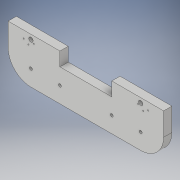
# Autodesk Inventor part: side drivetrain piece (8 wheel macanum)
Saved by Autodesk Inventor 2019 (Build 230136000, 136)
## iProperties
Created: 2019-04-20
Part Number: side drivetrain piece (8 wheel macanum)
Material: Generic
Document SubType Name: Modeling
Designer: Delta
Density: 1 g/cm^3
Appearance: Default
Author: Delta
Autodesk Inventor part; units mm, degrees
ref_plane "YZ Plane" through (0, 0, 0) normal (1, 0, 0) x (0, 1, 0)
ref_plane "XZ Plane" through (0, 0, 0) normal (0, 1, 0) x (-1, 0, 0)
ref_plane "XY Plane" through (0, 0, 0) normal (0, 0, 1) x (1, 0, 0)
sketch "Sketch1" plane through (0, 0, 0) normal (0, 0, 1) x (1, 0, 0)
  line L0 (-63.5, 0) -> (-368.3, 0)
  line L1 (-431.8, 63.5) -> (-431.8, 88.9)
  line L2 (-431.8, 88.9) -> (0, 88.9)
  line L3 (0, 88.9) -> (0, 63.5)
  arc A0 (-431.8, 63.5) -> (-368.3, 0) centre (-368.3, 63.5) ccw
  arc A1 (-63.5, 0) -> (0, 63.5) centre (-63.5, 63.5) ccw
  line L4 (-431.8, 88.9) -> (-287.8667, 88.9)
  line L5 (0, 88.9) -> (-143.9333, 88.9)
  point P0 (0, 0)
  point P1 (-431.8, 0)
  dimension "d0" = 431.8
  dimension "d1" = 88.9
  dimension "d2" = 63.5
  dimension "d3" = 63.5
  constraints: 12 end point, 4 point on circle, 4 point on line, 4 tangent, 3 horizontal, 2 centre point, 2 parallel, 1 perpendicular
  measures "d0" distance of L1.end L2.end
  measures "d1" distance of point (-431.8, 0) L1.end
  measures "d2" radius of A0
  measures "d3" radius of A1
extrude "Extrusion1" add sketch "Sketch1" along normal blind 23
sketch "Sketch2" plane through (0, 0, 23) normal (0, 0, 1) x (1, 0, 0)
  line L0 (-368.3, 0) -> (-63.5, 0) projected
  line L1 (0, 88.9) -> (-431.8, 88.9) projected
  line L2 (0, 63.5) -> (0, 88.9) projected
  line L3 (-431.8, 88.9) -> (-431.8, 63.5) projected
  point P0 (0, 0)
  point P1 (-368.3, 44.45)
  point P2 (-287.8667, 44.45)
  point P3 (-143.9333, 44.45)
  point P4 (-63.5, 44.45)
  dimension "d6" = 88.9
  dimension "d7" = 44.45
  dimension "d8" = 44.45
  dimension "d9" = 44.45
  dimension "d10" = 44.45
  dimension "d11" = 431.8
  dimension "d12" = 63.5
  dimension "d13" = 143.9333
  dimension "d14" = 143.9333
  dimension "d15" = 63.5
  measures "d6" distance between parallel lines of L0 L1
  measures "d7" distance from line of L1 point (-368.3, 44.45)
  measures "d8" distance from line of L1 point (-287.867, 44.45)
  measures "d9" distance from line of L1 point (-143.933, 44.45)
  measures "d10" distance from line of L1 point (-63.5, 44.45)
  measures "d11" distance between parallel lines of L2 L3
  measures "d12" distance from line of L3 point (-368.3, 44.45)
  measures "d13" distance from line of L3 point (-287.867, 44.45)
  measures "d14" distance from line of L2 point (-143.933, 44.45)
  measures "d15" distance from line of L2 point (-63.5, 44.45)
hole "Hole1" at (-368.3, 44.45, 23) at (-287.8667, 44.45, 23) at (-143.9333, 44.45, 23) at (-63.5, 44.45, 23) direction (0, 0, -1) diameter 7.9 end through all
sketch "Sketch3" plane through (-431.8, 88.9, 0) normal (0, 1, 0) x (1, 0, 0)
  line L0 (431.8, 0) -> (0, 0) projected
  line L1 (0, -23) -> (143.9333, -23)
  line L2 (143.9333, -23) -> (143.9333, 0)
  line L3 (143.9333, 0) -> (0, 0)
  line L4 (0, 0) -> (0, -23)
  line L5 (431.8, -23) -> (0, -23) projected
  line L6 (431.8, -23) -> (287.8667, -23)
  line L7 (287.8667, -23) -> (287.8667, 0)
  line L8 (287.8667, 0) -> (431.8, 0)
  line L9 (431.8, 0) -> (431.8, -23)
  dimension "d27" = 431.8
  dimension "d28" = 143.9333
  dimension "d29" = 143.9333
  constraints: 16 end point, 4 parallel, 2 horizontal, 2 perpendicular, 2 point on line
  measures "d27" distance of L0.start L0.end
  measures "d28" distance between parallel lines of L2 L4
  measures "d29" distance between parallel lines of L9 L7
extrude "Extrusion2" add sketch "Sketch3" along normal blind 38.1 contours L9 L5 L7 L0 | L2 L1 L4 L0
sketch "Sketch4" plane through (0, 0, 23) normal (0, 0, 1) x (1, 0, 0)
  line L0 (-143.9333, 88.9) -> (-143.9333, 127) projected
  line L1 (-287.8667, 88.9) -> (-287.8667, 127) projected
  line L2 (-143.9333, 127) -> (0, 127) projected
  line L3 (-431.8, 127) -> (-287.8667, 127) projected
  circle A0 centre (-368.3, 44.45) radius 3.95 projected
  circle A1 centre (-63.5, 44.45) radius 3.95 projected
  point P0 (0, 0)
  point P1 (-63.5, 114.3)
  point P2 (-368.3, 114.3)
  dimension "d32" = 38.1
  dimension "d33" = 38.1
  dimension "d34" = 12.7
  dimension "d35" = 12.7
  dimension "d38" = 0
  dimension "d39" = 0
  measures "d32" distance of L0.start L0.end
  measures "d33" distance of L1.start L1.end
  measures "d34" distance from line of L2 point (-63.5, 114.3)
  measures "d35" distance from line of L3 point (-368.3, 114.3)
  measures "d38" horizontal distance of A0.centre point (-368.3, 114.3)
  measures "d39" horizontal distance of A1.centre point (-63.5, 114.3)
hole "Hole2" at (-63.5, 114.3, 23) at (-368.3, 114.3, 23) direction (0, 0, -1) diameter 11.9888 end through all
sketch "Sketch5" plane through (0, 0, 23) normal (0, 0, 1) x (1, 0, 0)
  circle A0 centre (-368.3, 114.3) radius 5.9944 projected
  circle A1 centre (-63.5, 114.3) radius 5.9944 projected
  point P0 (0, 0)
  point P1 (-360.553, 107.8738)
  point P2 (-375.3104, 98.806)
  point P3 (-388.7216, 106.553)
  point P4 (-71.247, 107.8738)
  point P5 (-56.4896, 98.806)
  point P6 (-43.0784, 106.553)
  dimension "d47" = 7.747
  dimension "d48" = 6.4262
  dimension "d49" = 7.0104
  dimension "d50" = 15.494
  dimension "d51" = 20.4216
  dimension "d52" = 7.747
  dimension "d53" = 7.747
  dimension "d54" = 6.4262
  dimension "d55" = 15.494
  dimension "d56" = 7.0104
  dimension "d57" = 7.747
  dimension "d58" = 20.4216
  measures "d47" horizontal distance of point (-360.553, 107.874) A0.centre
  measures "d48" vertical distance of point (-360.553, 107.874) A0.centre
  measures "d49" horizontal distance of point (-375.31, 98.806) A0.centre
  measures "d50" vertical distance of point (-375.31, 98.806) A0.centre
  measures "d51" horizontal distance of A0.centre point (-388.722, 106.553)
  measures "d52" vertical distance of A0.centre point (-388.722, 106.553)
  measures "d53" horizontal distance of A1.centre point (-71.247, 107.874)
  measures "d54" vertical distance of A1.centre point (-71.247, 107.874)
  measures "d55" vertical distance of point (-56.49, 98.806) A1.centre
  measures "d56" horizontal distance of A1.centre point (-56.49, 98.806)
  measures "d57" vertical distance of A1.centre point (-43.078, 106.553)
  measures "d58" horizontal distance of A1.centre point (-43.078, 106.553)
hole "Hole3" at (-360.553, 107.8738, 23) at (-375.3104, 98.806, 23) at (-388.7216, 106.553, 23) at (-71.247, 107.8738, 23) at (-56.4896, 98.806, 23) at (-43.0784, 106.553, 23) direction (0, 0, -1) diameter 3.175 end through all
equation "\"d7\" = 0.5 * d6"
equation "\"d8\" = 0.5 * d6"
equation "\"d9\" = 0.5 * d6"
equation "\"d10\" = 0.5 * d6"
equation "\"d13\" = 0.333333 * d11"
equation "\"d14\" = d13"
equation "\"d15\" = d12"
equation "\"d28\" = 0.333333 * d27"
equation "\"d29\" = d28"
equation "\"d34\" = 0.333333 * d32"
equation "\"d35\" = 0.333333 * d33"
equation "\"d53\" = d47"
equation "\"d54\" = d48"
equation "\"d55\" = d50"
equation "\"d56\" = d49"
equation "\"d57\" = d52"
equation "\"d58\" = d51"
body "Solid1"
